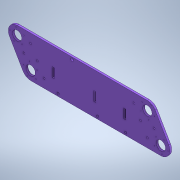
# Autodesk Inventor part: stenka
Saved by Autodesk Inventor 2020 (Build 240168000, 168)
## iProperties
Created: 2022-01-12
Part Number: stenka
Material: Типовые
Document SubType Name: Modeling
Designer: solidworks
Density: 1 g/cm^3
Appearance: По умолчанию
Author: solidworks
Autodesk Inventor part; units mm, degrees
ref_plane "YZ Plane" through (0, 0, 0) normal (1, 0, 0) x (0, 1, 0)
ref_plane "XZ Plane" through (0, 0, 0) normal (0, 1, 0) x (-1, 0, 0)
ref_plane "XY Plane" through (0, 0, 0) normal (0, 0, 1) x (1, 0, 0)
sketch "Эскиз1" plane through (0, 0, 0) normal (0, 0, 1) x (1, 0, 0)
  line L0 (0, 0) -> (351.5171, 0) construction
  line L1 (28.8675, 50) -> (528.8675, 50) construction
  line L2 (528.8675, 50) -> (528.8675, 200) construction
  circle A0 centre (-28.8675, 150) radius 20
  circle A1 centre (28.8675, 50) radius 20
  circle A2 centre (586.6025, 50) radius 20
  circle A3 centre (528.8675, 150) radius 20
  circle A4 centre (528.8675, 150) radius 50 construction
  circle A5 centre (28.8675, 50) radius 50 construction
  line L3 (478.8675, 150) -> (478.8675, 60) construction
  line L4 (78.8675, 60) -> (78.8675, 200) construction
  line L5 (478.8675, 150) -> (478.8675, 200) construction
  line L6 (-86.0463, 60) -> (78.8675, 60) construction
  arc A6 (561.7765, 169) -> (528.8675, 188) centre (528.8675, 150) ccw
  arc A7 (586.6025, 12) -> (619.5115, 69) centre (586.6025, 50) ccw
  arc A8 (-28.8675, 188) -> (-61.7765, 131) centre (-28.8675, 150) ccw
  arc A9 (-4.0415, 31) -> (28.8675, 12) centre (28.8675, 50) ccw
  line L7 (-61.7765, 131) -> (-4.0415, 31)
  line L8 (478.8675, 60) -> (623.2631, 60) construction
  line L9 (635.5923, 60) -> (638.5641, 60) construction
  line L10 (561.7765, 169) -> (619.5115, 69)
  circle A10 centre (-28.8675, 150) radius 50 construction
  line L11 (-45.5421, 103.966) -> (-45.7799, 104.0432) construction
  arc A11 (-2.1023, 179.4126) -> (3.5169, 179.4126) centre (0.7073, 183.2797) ccw construction
  arc A12 (-9.1654, 184.5442) -> (-2.1023, 179.4126) centre (-2.2483, 186.6382) ccw construction
  arc A13 (-10.9018, 189.8884) -> (-9.1654, 184.5442) centre (-6.3557, 188.4113) ccw construction
  line L12 (10.7754, 48.5676) -> (10.8465, 48.7864)
  line L13 (8.5834, 183.0936) -> (14.1794, 175.3914)
  line L14 (49.7439, -4.7602) -> (49.7729, -4.7602) construction
  line L15 (49.7504, 4.7602) -> (49.7729, 4.7602) construction
  line L16 (49.7504, 4.7602) -> (49.7504, 4.9902) construction
  line L17 (8.5834, 183.0936) -> (3.5169, 179.4126) construction
  line L18 (-10.9018, 189.8884) -> (-8.9686, 195.8382) construction
  line L19 (-18.0211, 198.7864) -> (-8.9666, 195.8444)
  line L20 (-18.0211, 198.7864) -> (-19.9563, 192.8304) construction
  arc A14 (-24.5023, 189.5275) -> (-19.9563, 192.8304) centre (-24.5023, 194.3075) ccw construction
  arc A15 (-33.2327, 189.5275) -> (-24.5023, 189.5275) centre (-28.8675, 195.2874) ccw construction
  arc A16 (-37.7787, 192.8304) -> (-33.2327, 189.5275) centre (-33.2327, 194.3075) ccw construction
  line L21 (-37.7787, 192.8304) -> (-39.712, 198.7802) construction
  line L22 (-48.7685, 195.8444) -> (-39.714, 198.7864)
  line L23 (-48.7685, 195.8444) -> (-46.8332, 189.8884) construction
  arc A17 (-48.5697, 184.5442) -> (-46.8332, 189.8884) centre (-51.3793, 188.4113) ccw construction
  arc A18 (-55.6327, 179.4126) -> (-48.5697, 184.5442) centre (-55.4868, 186.6382) ccw construction
  arc A19 (-61.2519, 179.4126) -> (-55.6327, 179.4126) centre (-58.4423, 183.2797) ccw construction
  line L24 (-61.2519, 179.4126) -> (-66.3131, 183.0898) construction
  line L25 (-71.9144, 175.3914) -> (-66.3184, 183.0936)
  line L26 (-71.9144, 175.3914) -> (-66.8479, 171.7104) construction
  arc A20 (-65.1114, 166.3662) -> (-66.8479, 171.7104) centre (-69.6575, 167.8433) ccw construction
  arc A21 (-67.8093, 158.0631) -> (-65.1114, 166.3662) centre (-71.9383, 163.9946) ccw construction
  arc A22 (-72.3553, 154.7602) -> (-67.8093, 158.0631) centre (-72.3553, 159.5402) ccw construction
  line L27 (-72.3553, 154.7602) -> (-78.6114, 154.7602) construction
  line L28 (-78.6179, 145.2398) -> (-78.6179, 154.7602)
  line L29 (-78.6179, 145.2398) -> (-72.3553, 145.2398) construction
  arc A23 (-67.8093, 141.9369) -> (-72.3553, 145.2398) centre (-72.3553, 140.4598) ccw construction
  arc A24 (-65.1114, 133.6338) -> (-67.8093, 141.9369) centre (-71.9383, 136.0054) ccw construction
  arc A25 (-66.8479, 128.2896) -> (-65.1114, 133.6338) centre (-69.6575, 132.1567) ccw construction
  line L30 (-66.8479, 128.2896) -> (-71.9091, 124.6124) construction
  line L31 (-66.3184, 116.9064) -> (-71.9144, 124.6086)
  line L32 (-66.3184, 116.9064) -> (-61.2519, 120.5874) construction
  arc A26 (-55.6327, 120.5874) -> (-61.2519, 120.5874) centre (-58.4423, 116.7203) ccw construction
  arc A27 (-48.5697, 115.4558) -> (-55.6327, 120.5874) centre (-55.4868, 113.3618) ccw construction
  arc A28 (-46.8332, 110.1116) -> (-48.5697, 115.4558) centre (-51.3793, 111.5887) ccw construction
  line L33 (-46.8332, 110.1116) -> (-48.7665, 104.1618) construction
  line L34 (-39.714, 101.2136) -> (-48.7685, 104.1556)
  line L35 (-39.714, 101.2136) -> (-37.7787, 107.1696) construction
  arc A29 (-33.2327, 110.4725) -> (-37.7787, 107.1696) centre (-33.2327, 105.6925) ccw construction
  arc A30 (-24.5023, 110.4725) -> (-33.2327, 110.4725) centre (-28.8675, 104.7126) ccw construction
  arc A31 (-19.9563, 107.1696) -> (-24.5023, 110.4725) centre (-24.5023, 105.6925) ccw construction
  line L36 (-19.9563, 107.1696) -> (-18.0231, 101.2198) construction
  line L37 (-8.9666, 104.1556) -> (-18.0211, 101.2136)
  line L38 (-8.9666, 104.1556) -> (-10.9018, 110.1116) construction
  arc A32 (-9.1654, 115.4558) -> (-10.9018, 110.1116) centre (-6.3557, 111.5887) ccw construction
  arc A33 (-2.1023, 120.5874) -> (-9.1654, 115.4558) centre (-2.2483, 113.3618) ccw construction
  arc A34 (3.5169, 120.5874) -> (-2.1023, 120.5874) centre (0.7073, 116.7203) ccw construction
  line L39 (3.5169, 120.5874) -> (8.5781, 116.9102) construction
  line L40 (14.1794, 124.6086) -> (8.5834, 116.9064)
  line L41 (14.1794, 124.6086) -> (9.1129, 128.2896) construction
  arc A35 (7.3764, 133.6338) -> (9.1129, 128.2896) centre (11.9225, 132.1567) ccw construction
  arc A36 (10.0743, 141.9369) -> (7.3764, 133.6338) centre (14.2033, 136.0054) ccw construction
  arc A37 (14.6203, 145.2398) -> (10.0743, 141.9369) centre (14.6203, 140.4598) ccw construction
  line L42 (14.6203, 145.2398) -> (20.8763, 145.2398) construction
  line L43 (20.8828, 154.7602) -> (20.8828, 145.2398)
  line L44 (20.8828, 154.7602) -> (14.6203, 154.7602) construction
  arc A38 (10.0743, 158.0631) -> (14.6203, 154.7602) centre (14.6203, 159.5402) ccw construction
  arc A39 (7.3764, 166.3662) -> (10.0743, 158.0631) centre (14.2033, 163.9946) ccw construction
  arc A40 (9.1129, 171.7104) -> (7.3764, 166.3662) centre (11.9225, 167.8433) ccw construction
  line L45 (9.1129, 171.7104) -> (14.1741, 175.3876) construction
  line L46 (508.9665, 195.8444) -> (510.9018, 189.8884) construction
  arc A41 (509.1653, 184.5442) -> (510.9018, 189.8884) centre (506.3557, 188.4113) ccw construction
  arc A42 (502.1023, 179.4126) -> (509.1653, 184.5442) centre (502.2482, 186.6382) ccw construction
  arc A43 (496.4831, 179.4126) -> (502.1023, 179.4126) centre (499.2927, 183.2797) ccw construction
  line L47 (485.8206, 175.3914) -> (491.4166, 183.0936)
  line L48 (496.4831, 179.4126) -> (491.4219, 183.0898) construction
  line L49 (508.9665, 195.8444) -> (518.021, 198.7864)
  line L50 (519.9563, 192.8304) -> (518.023, 198.7802) construction
  arc A44 (519.9563, 192.8304) -> (524.5023, 189.5275) centre (524.5023, 194.3075) ccw construction
  arc A45 (524.5023, 189.5275) -> (533.2327, 189.5275) centre (528.8675, 195.2874) ccw construction
  arc A46 (533.2327, 189.5275) -> (537.7787, 192.8304) centre (533.2327, 194.3075) ccw construction
  line L51 (539.7139, 198.7864) -> (537.7787, 192.8304) construction
  line L52 (539.7139, 198.7864) -> (548.7684, 195.8444)
  line L53 (546.8332, 189.8884) -> (548.7664, 195.8382) construction
  arc A47 (546.8332, 189.8884) -> (548.5696, 184.5442) centre (551.3793, 188.4113) ccw construction
  arc A48 (548.5696, 184.5442) -> (555.6327, 179.4126) centre (555.4867, 186.6382) ccw construction
  arc A49 (555.6327, 179.4126) -> (561.2519, 179.4126) centre (558.4423, 183.2797) ccw construction
  line L54 (566.3184, 183.0936) -> (561.2519, 179.4126) construction
  line L55 (566.3184, 183.0936) -> (571.9144, 175.3914)
  line L56 (566.8479, 171.7104) -> (571.9091, 175.3876) construction
  arc A50 (566.8479, 171.7104) -> (565.1114, 166.3662) centre (569.6575, 167.8433) ccw construction
  arc A51 (565.1114, 166.3662) -> (567.8093, 158.0631) centre (571.9383, 163.9946) ccw construction
  arc A52 (567.8093, 158.0631) -> (572.3553, 154.7602) centre (572.3553, 159.5402) ccw construction
  line L57 (578.6178, 154.7602) -> (572.3553, 154.7602) construction
  line L58 (578.6178, 154.7602) -> (578.6178, 145.2398)
  line L59 (572.3553, 145.2398) -> (578.6113, 145.2398) construction
  arc A53 (572.3553, 145.2398) -> (567.8093, 141.9369) centre (572.3553, 140.4598) ccw construction
  arc A54 (567.8093, 141.9369) -> (565.1114, 133.6338) centre (571.9383, 136.0054) ccw construction
  arc A55 (565.1114, 133.6338) -> (566.8479, 128.2896) centre (569.6575, 132.1567) ccw construction
  line L60 (571.9144, 124.6086) -> (566.8479, 128.2896) construction
  line L61 (571.9144, 124.6086) -> (566.3184, 116.9064)
  line L62 (561.2519, 120.5874) -> (566.3131, 116.9102) construction
  arc A56 (561.2519, 120.5874) -> (555.6327, 120.5874) centre (558.4423, 116.7203) ccw construction
  arc A57 (555.6327, 120.5874) -> (548.5696, 115.4558) centre (555.4867, 113.3618) ccw construction
  arc A58 (548.5696, 115.4558) -> (546.8332, 110.1116) centre (551.3793, 111.5887) ccw construction
  line L63 (548.7684, 104.1556) -> (546.8332, 110.1116) construction
  line L64 (548.7684, 104.1556) -> (539.7139, 101.2136)
  line L65 (537.7787, 107.1696) -> (539.7119, 101.2198) construction
  arc A59 (537.7787, 107.1696) -> (533.2327, 110.4725) centre (533.2327, 105.6925) ccw construction
  arc A60 (533.2327, 110.4725) -> (524.5023, 110.4725) centre (528.8675, 104.7126) ccw construction
  arc A61 (524.5023, 110.4725) -> (519.9563, 107.1696) centre (524.5023, 105.6925) ccw construction
  line L66 (518.021, 101.2136) -> (519.9563, 107.1696) construction
  line L67 (518.021, 101.2136) -> (508.9665, 104.1556)
  line L68 (510.9018, 110.1116) -> (508.9685, 104.1618) construction
  arc A62 (510.9018, 110.1116) -> (509.1653, 115.4558) centre (506.3557, 111.5887) ccw construction
  arc A63 (509.1653, 115.4558) -> (502.1023, 120.5874) centre (502.2482, 113.3618) ccw construction
  arc A64 (502.1023, 120.5874) -> (496.4831, 120.5874) centre (499.2927, 116.7203) ccw construction
  line L69 (491.4166, 116.9064) -> (496.4831, 120.5874) construction
  line L70 (491.4166, 116.9064) -> (485.8206, 124.6086)
  line L71 (490.8871, 128.2896) -> (485.8259, 124.6124) construction
  arc A65 (490.8871, 128.2896) -> (492.6236, 133.6338) centre (488.0775, 132.1567) ccw construction
  arc A66 (492.6236, 133.6338) -> (489.9257, 141.9369) centre (485.7967, 136.0054) ccw construction
  arc A67 (489.9257, 141.9369) -> (485.3797, 145.2398) centre (485.3797, 140.4598) ccw construction
  line L72 (479.1171, 145.2398) -> (485.3797, 145.2398) construction
  line L73 (479.1171, 145.2398) -> (479.1171, 154.7602)
  line L74 (485.3797, 154.7602) -> (479.1236, 154.7602) construction
  arc A68 (485.3797, 154.7602) -> (489.9257, 158.0631) centre (485.3797, 159.5402) ccw construction
  arc A69 (489.9257, 158.0631) -> (492.6236, 166.3662) centre (485.7967, 163.9946) ccw construction
  arc A70 (492.6236, 166.3662) -> (490.8871, 171.7104) centre (488.0775, 167.8433) ccw construction
  line L75 (485.8206, 175.3914) -> (490.8871, 171.7104) construction
  circle A71 centre (528.8675, 150) radius 50 construction
  line L76 (528.8675, 188) -> (-28.8675, 188)
  line L77 (586.6025, 12) -> (28.8675, 12)
  line L78 (435.8675, 60) -> (121.8675, 60) construction
  line L79 (478.8675, 60) -> (435.8675, 60) construction
  line L80 (78.8675, 60) -> (121.8675, 60) construction
  line L81 (121.8675, 70) -> (435.8675, 70) construction
  line L82 (435.8675, 70) -> (427.8675, 70)
  line L83 (427.8675, 110) -> (435.8675, 110)
  line L84 (121.8675, 70) -> (129.8675, 70)
  line L85 (129.8675, 110) -> (121.8675, 110)
  line L86 (427.8675, 70) -> (307.8675, 70) construction
  line L87 (307.8675, 70) -> (299.8675, 70)
  line L88 (299.8675, 110) -> (307.8675, 110)
  line L89 (121.8675, 110) -> (121.3675, 110)
  line L90 (121.3675, 110) -> (121.3675, 70)
  line L91 (121.3675, 70) -> (121.8675, 70)
  line L92 (129.8675, 70) -> (130.3675, 70)
  line L93 (130.3675, 70) -> (130.3675, 110)
  line L94 (130.3675, 110) -> (129.8675, 110)
  line L95 (299.8675, 110) -> (299.3675, 110)
  line L96 (299.3675, 110) -> (299.3675, 70)
  line L97 (299.8675, 70) -> (299.3675, 70)
  line L98 (307.8675, 70) -> (308.3675, 70)
  line L99 (308.3675, 70) -> (308.3675, 110)
  line L100 (308.3675, 110) -> (307.8675, 110)
  line L101 (435.8675, 70) -> (436.3675, 70)
  line L102 (436.3675, 70) -> (436.3675, 110)
  line L103 (436.3675, 110) -> (435.8675, 110)
  line L104 (427.8675, 110) -> (427.3675, 110)
  line L105 (427.3675, 110) -> (427.3675, 70)
  line L106 (427.8675, 70) -> (427.3675, 70)
  dimension "d44" = 360
  dimension "d46" = 360
  dimension "d9" = 40
  dimension "d10" = 40
  dimension "d11" = 40
  dimension "d12" = 40
  dimension "d29" = 76
  dimension "d30" = 76
  dimension "d31" = 76
  dimension "d35" = 100
  dimension "d49" = 360
  dimension "d53" = 557.735
  dimension "d58" = 549.0046
  dimension "d59" = 314
  dimension "d60" = 10
  dimension "d61" = 8
  dimension "d62" = 40
  dimension "d63" = 8
  dimension "d64" = 40
  dimension "d69" = 8
  dimension "d71" = 0.5
  dimension "d72" = 0.5
  dimension "d73" = 0.5
  dimension "d74" = 0.5
  dimension "d75" = 0.5
  dimension "d76" = 0.5
  constraints: 214 end point, 129 point on circle, 71 centre point, 14 horizontal, 13 perpendicular, 13 point on line, 7 coincident, 6 parallel, 5 tangent, 3 collinear, 3 vertical, 1 horizontal alignment, 327 other
  measures "d9" diameter of A0
  measures "d10" diameter of A1
  measures "d11" diameter of A2
  measures "d12" diameter of A3
  measures "d29" diameter of A6
  measures "d30" diameter of A7
  measures "d31" diameter of A8
  measures "d35" diameter of A10
  measures "d53" distance of L23.end L46.end
  measures "d58" distance of A44.centre A14.centre
  measures "d59" distance of L78.start L78.end
  measures "d60" distance between parallel lines of L81 L78
  measures "d61" distance of L83.start L83.end
  measures "d62" distance of L82.end L83.start
  measures "d63" distance of L85.end L85.start
  measures "d64" distance of L85.start L84.end
  measures "d69" distance of L88.start L88.end
  measures "d71" distance of L85.end L89.end
  measures "d72" distance of L84.end L92.end
  measures "d73" distance of L88.start L95.end
  measures "d74" distance of L86.end L98.end
  measures "d75" distance of L81.end L101.end
  measures "d76" distance of L83.start L104.end
extrude "Выдавливание2" add sketch "Эскиз1" along normal blind 8
sketch "Эскиз2" plane through (0, 0, 8) normal (0, 0, 1) x (1, 0, 0)
  circle A0 centre (28.8675, 150) radius 4 projected
  circle A1 centre (-1.4222, 163.9841) radius 2 projected
  circle A2 centre (-7.0868, 128.2193) radius 2 projected
  circle A3 centre (-42.8516, 122.5547) radius 2 projected
  circle A4 centre (-59.2909, 154.8186) radius 2 projected
  circle A5 centre (-33.6861, 180.4234) radius 2 projected
  circle A6 centre (57.735, 100) radius 4 projected
  circle A7 centre (86.6025, 50) radius 4 projected
  circle A8 centre (56.3128, 63.9841) radius 2 projected
  circle A9 centre (50.6482, 28.2193) radius 2 projected
  circle A10 centre (14.8834, 22.5547) radius 2 projected
  circle A11 centre (-1.5559, 54.8186) radius 2 projected
  circle A12 centre (24.0489, 80.4234) radius 2 projected
  circle A13 centre (559.1572, 36.0159) radius 2 projected
  circle A14 centre (564.8218, 71.7807) radius 2 projected
  circle A15 centre (559.1572, 36.0159) radius 2 projected
  circle A16 centre (600.5866, 77.4453) radius 2 projected
  circle A17 centre (617.0259, 45.1814) radius 2 projected
  circle A18 centre (564.8218, 71.7807) radius 2 projected
  circle A19 centre (591.4211, 19.5766) radius 2 projected
  circle A20 centre (617.0259, 45.1814) radius 2 projected
  circle A21 centre (507.0868, 171.7807) radius 2 projected
  circle A22 centre (542.8516, 177.4453) radius 2 projected
  circle A23 centre (559.2909, 145.1814) radius 2 projected
  circle A24 centre (533.6861, 119.5766) radius 2 projected
  circle A25 centre (501.4222, 136.0159) radius 2 projected
  circle A26 centre (557.735, 100) radius 4 projected
  circle A27 centre (528.8675, 50) radius 4 projected
  circle A28 centre (500, 100) radius 4 projected
  circle A29 centre (471.1325, 150) radius 4 projected
  circle A30 centre (0, 100) radius 4 projected
  circle A31 centre (146.2756, 23) radius 5
  circle A32 centre (436.2756, 23) radius 5
  circle A33 centre (316.2756, 23) radius 5
  line L0 (28.8675, 12) -> (586.6025, 12) projected
  circle A34 centre (205.8026, 178) radius 6
  line L1 (528.8675, 188) -> (-28.8675, 188) projected
  point P0 (0, 0)
  dimension "d77" = 10
  dimension "d78" = 10
  dimension "d79" = 10
  dimension "d80" = 11
  dimension "d81" = 11
  dimension "d82" = 11
  dimension "d83" = 120
  dimension "d84" = 170
  dimension "d85" = 12
  dimension "d86" = 10
  constraints: 4 centre point
  measures "d77" diameter of A31
  measures "d78" diameter of A32
  measures "d79" diameter of A33
  measures "d80" distance from line of L0 A32.centre
  measures "d81" distance from line of L0 A33.centre
  measures "d82" distance from line of L0 A31.centre
  measures "d83" distance of A33.centre A32.centre
  measures "d84" distance of A31.centre A33.centre
  measures "d85" diameter of A34
  measures "d86" distance from line of L1 A34.centre
extrude "Выдавливание3" cut sketch "Эскиз2" against normal through all
